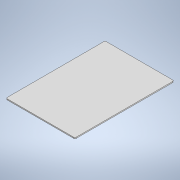
# Autodesk Inventor part: 演講稿
Saved by Autodesk Inventor 2021 (Build 250183000, 183)
## iProperties
Created: 2023-03-01
Part Number: 演講稿
Material: 一般
Document SubType Name: Modeling
Designer: brian
Density: 1 g/cm^3
Appearance: 預設
Author: brian
Autodesk Inventor part; units mm, degrees
ref_plane "YZ Plane" through (0, 0, 0) normal (1, 0, 0) x (0, 1, 0)
ref_plane "XZ Plane" through (0, 0, 0) normal (0, 1, 0) x (-1, 0, 0)
ref_plane "XY Plane" through (0, 0, 0) normal (0, 0, 1) x (1, 0, 0)
sketch "草圖1" plane through (0, 0, 0) normal (0, 1, 0) x (-1, 0, 0)
  line L0 (-160, 230) -> (160, 230)
  line L1 (160, 230) -> (160, -230)
  line L2 (160, -230) -> (-160, -230)
  line L3 (-160, -230) -> (-160, 230)
  line L4 (-160, 230) -> (160, -230) construction
  line L5 (160, 230) -> (-160, -230) construction
  point P0 (0, 0)
  dimension "d0" = 320
  dimension "d1" = 460
  constraints: 12 end point, 2 midpoint, 2 parallel, 1 horizontal, 1 perpendicular
  measures "d0" distance of L1.end L2.end
  measures "d1" distance of L0.end L1.end
extrude "擠出1" add sketch "草圖1" along normal blind 5
fillet "圓角1" radius 5 4 edges at (160, 2.5, 230) (160, 2.5, -230) (-160, 2.5, -230) (-160, 2.5, 230)
